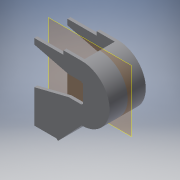
# Autodesk Inventor part: casco-salida-0,1
Saved by Autodesk Inventor 2016 (Build 200138000, 138)
## iProperties
Created: 2015-03-24
Part Number: casco-salida-0,1
Material: Generic
Document SubType Name: Modeling
Designer: pc
Density: 1 g/cm^3
Appearance: Default
Author: pc
Autodesk Inventor part; units mm, degrees
ref_plane "YZ Plane" through (0, 0, 0) normal (1, 0, 0) x (0, 1, 0)
ref_plane "XZ Plane" through (0, 0, 0) normal (0, 1, 0) x (-1, 0, 0)
ref_plane "XY Plane" through (0, 0, 0) normal (0, 0, 1) x (1, 0, 0)
sketch "Sketch1" plane through (0, 0, 0) normal (1, 0, 0) x (0, 1, 0)
  line L0 (0, -6.7778) -> (70, -6.7778)
  line L1 (70, -6.7778) -> (70, -64.7778)
  line L2 (0, -64.7778) -> (0, -6.7778)
  line L3 (77, -64.7778) -> (77, 0.2222)
  line L4 (77, 0.2222) -> (-7, 0.2222)
  line L5 (-7, 0.2222) -> (-7, -64.7778)
  line L6 (-7, -64.7778) -> (77, -64.7778)
  point P0 (0, 0)
  dimension "d2" = 7
  dimension "d3" = 65
  dimension "d5" = 58
  dimension "d6" = 84
  constraints: 14 end point, 3 parallel, 2 perpendicular, 2 point on line, 1 horizontal
  measures "d2" distance between parallel lines of L1 L3
  measures "d3" distance of L4.end L5.end
  measures "d5" distance between parallel lines of L0 L6
  measures "d6" distance of L3.end L4.end
revolve "Revolution1" add sketch "Sketch1" angle 180 about axis through (0, -7, -64.7778) along (0, 1, 0) contours L2 L6 L5 L4 L3 L1 L0
sketch "Sketch2" plane through (0, -7, 0.2222) normal (-1, 0, 0) x (0, 0, 1)
  line L0 (0, 0) -> (-130, 0) projected
  line L1 (0, 0) -> (-130, 0) projected
  line L2 (0, 84) -> (0, 0) projected
  line L3 (0, 84) -> (-130, 84) projected
  line L4 (-130, 84) -> (-130, 0) projected
  line L5 (-7, 7) -> (-123, 7) projected
  line L6 (-123, 7) -> (-123, 77) projected
  line L7 (-7, 77) -> (-123, 77) projected
  line L8 (-7, 7) -> (-7, 77) projected
  line L9 (0, 0) -> (-42, 0)
  line L10 (-42, 0) -> (-42, 7)
  line L11 (-42, 7) -> (0, 7)
  line L12 (0, 7) -> (0, 0)
  line L13 (0, 0) -> (0, 42)
  line L14 (0, 77) -> (0, 84)
  point P0 (-0.2222, 7)
  point P1 (-130, 84)
  dimension "d7" = 42
  constraints: 12 end point, 2 parallel, 1 horizontal, 1 perpendicular, 1 point on line
  measures "d7" distance between parallel lines of L10 L2
extrude "Extrusion1" add sketch "Sketch2" along normal blind 110 contours L0 L10 L5 L11 L2
sketch "Sketch3" plane through (-110, -7, 0.2222) normal (0, -1, 0) x (1, 0, 0)
  line L0 (110, -42) -> (110, -130) projected
  arc A0 (110, -130) -> (110, 0) centre (110, -65) ccw projected
  line L1 (110, 0) -> (0, 0) projected
  line L2 (0, -42) -> (0, 0) projected
  line L3 (110, -42) -> (0, -42) projected
  line L4 (110, 0) -> (0, 0)
  line L5 (110, 0) -> (0, 0) projected
  line L6 (110, -42) -> (80, -42)
  line L7 (110, -42) -> (0, -42) projected
  line L8 (0, -42) -> (0, 0) projected
  line L9 (80, -42) -> (0, -22.0538)
  point P0 (110, -0.2222)
  dimension "d11" = 30
  dimension "d13" = 14
  constraints: 6 end point, 3 point on line
  measures "d11" distance of L0.start L6.end
  measures "d13" angle of L9 L3
extrude "Extrusion2" cut sketch "Sketch3" against normal through all contours L3 L2 L9
ref_plane "Work Plane1" through (-110, 35, 0.2222) normal (0, -1, 0) x (1, 0, 0)
mirror "Mirror1" about plane through (-110, 35, 0.2222) normal (0, -1, 0) of "Extrusion1", "Extrusion2"
sketch "Sketch4" plane through (-110, -7, 0.2222) normal (0, -1, 0) x (1, 0, 0)
  line L0 (0, -22.0538) -> (80, -42) projected
  line L1 (110, -42) -> (80, -42) projected
  line L2 (110, -42) -> (110, -130) projected
  arc A0 (110, -130) -> (110, 0) centre (110, -65) ccw projected
  line L3 (110, 0) -> (0, 0) projected
  line L4 (0, -22.0538) -> (0, 0) projected
  line L5 (110, -84) -> (110, -42)
  line L6 (113, -65) -> (113, -44)
  line L7 (113, -44) -> (110, -44)
  line L8 (110, -44) -> (110, -65)
  line L9 (110, -86) -> (110, -42)
  line L10 (113, -65) -> (113, -86)
  line L11 (113, -86) -> (110, -86)
  line L12 (110, -44) -> (110, -86)
  line L13 (110, -42) -> (110, -123) projected
  point P0 (110, -0.2222)
  point P1 (110, -88)
  dimension "d17" = 21
  dimension "d18" = 3
  constraints: 16 end point, 1 collinear, 1 parallel, 1 point on line
  measures "d17" distance of L6.start L6.end
  measures "d18" distance of L8.end L6.start
extrude "Extrusion3" cut sketch "Sketch4" against normal through all contours L7 L6 L10 L11 L2
sketch "Sketch5" plane through (-110, -7, 0.2222) normal (0, -1, 0) x (1, 0, 0)
  line L0 (113, -86) -> (110, -86) projected
  line L1 (110, -86) -> (110, -130) projected
  arc A0 (110, -130) -> (110, 0) centre (110, -65) ccw projected
  line L2 (110, 0) -> (0, 0) projected
  line L3 (0, -22.0538) -> (0, 0) projected
  line L4 (0, -22.0538) -> (80, -42) projected
  line L5 (110, -42) -> (80, -42) projected
  line L6 (110, -42) -> (110, -44) projected
  line L7 (110, -44) -> (113, -44) projected
  line L8 (113, -44) -> (113, -86) projected
  line L9 (110, -130) -> (55.2127, -188.2954)
  arc A1 (110, -123) -> (110, -7) centre (110, -65) ccw projected
  line L10 (110, -123) -> (51.7311, -185)
  line L11 (51.7311, -185) -> (55.2244, -188.283)
  point P0 (110, -0.2222)
  dimension "d21" = 80
  constraints: 6 end point, 1 parallel, 1 perpendicular, 1 point on line
  measures "d21" distance of L1.end L9.end
extrude "Extrusion4" add sketch "Sketch5" against normal blind 84 contours L1 L9 L11 L10
sketch "Sketch6" plane through (-110, -7, 0.2222) normal (0, -1, 0) x (1, 0, 0)
  line L0 (113, -86) -> (110, -86) projected
  line L1 (110, -86) -> (110, -123) projected
  line L2 (110, -123) -> (51.7311, -185) projected
  line L3 (51.7311, -185) -> (55.2244, -188.283) projected
  line L4 (55.2244, -188.283) -> (110, -130) projected
  arc A0 (110, -130) -> (110, 0) centre (110, -65) ccw projected
  line L5 (110, 0) -> (0, 0) projected
  line L6 (0, -22.0538) -> (0, 0) projected
  line L7 (0, -22.0538) -> (80, -42) projected
  line L8 (110, -42) -> (80, -42) projected
  line L9 (110, -42) -> (110, -44) projected
  line L10 (110, -44) -> (113, -44) projected
  line L11 (113, -44) -> (113, -86) projected
  line L12 (110, -65) -> (80, -65)
  line L13 (0, -107.9462) -> (80, -88)
  line L14 (110, -88) -> (80, -88)
  line L15 (0, -107.9462) -> (0, -185)
  line L16 (0, -185) -> (51.7311, -185)
  line L17 (110, -88) -> (110, -123)
  line L18 (110, -123) -> (51.7311, -185)
  point P0 (110, -0.2222)
  constraints: 14 end point, 3 symmetric about line, 2 vertical, 1 horizontal, 1 perpendicular
extrude "Extrusion5" add sketch "Sketch6" against normal blind 7 contours L1 L2 L16 L15 L13 L14
mirror "Mirror2" about plane through (-110, 35, 0.2222) normal (0, -1, 0) of "Extrusion5"
sketch "Sketch7" plane through (-110, 77, 0.2222) normal (0, 1, 0) x (1, 0, 0)
  line L0 (0, 0) -> (68, 0)
  line L1 (110, 0) -> (0, 0) projected
  line L2 (68, 0) -> (68, 9)
  line L3 (68, 9) -> (0, 9)
  line L4 (0, 9) -> (0, 0)
  point P0 (110, 0.2222)
  dimension "d26" = 68
  dimension "d27" = 9
  constraints: 8 end point, 3 perpendicular, 1 point on line
  measures "d26" distance of L0.start L0.end
  measures "d27" distance of L0.end L2.end
extrude "Extrusion6" cut sketch "Sketch7" against normal blind 84
body "Solid1"
